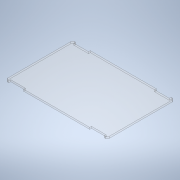
# Autodesk Inventor part: roof
Saved by Autodesk Inventor 2020 (Build 240168000, 168)
## iProperties
Created: 2020-03-02
Part Number: roof
Material: Polycarbonate, Clear
Document SubType Name: Modeling
Designer: n10208577
Density: 1.2 g/cm^3
Appearance: Polycarbonate - Clear
Author: n10208577
Autodesk Inventor part; units mm, degrees
ref_plane "YZ Plane" through (0, 0, 0) normal (1, 0, 0) x (0, 1, 0)
ref_plane "XZ Plane" through (0, 0, 0) normal (0, 1, 0) x (-1, 0, 0)
ref_plane "XY Plane" through (0, 0, 0) normal (0, 0, 1) x (1, 0, 0)
sketch "Sketch1" plane through (0, 0, 0) normal (0, 1, 0) x (-1, 0, 0)
  line L0 (25.1331, -7.9898) -> (138.1331, -7.9898)
  line L1 (-4.8669, 103.0102) -> (-4.8669, -4.9898)
  arc A0 (-4.8669, -4.9898) -> (-1.8669, -7.9898) centre (-1.8669, -4.9898) ccw
  line L2 (0.1331, -7.9898) -> (0.1331, -4.9898)
  line L3 (0.1331, -4.9898) -> (25.1331, -4.9898)
  line L4 (25.1331, -4.9898) -> (25.1331, -7.9898)
  line L5 (165.1331, -7.9898) -> (163.1331, -7.9898)
  line L6 (163.1331, -7.9898) -> (163.1331, -4.9898)
  line L7 (163.1331, -4.9898) -> (138.1331, -4.9898)
  line L8 (138.1331, -4.9898) -> (138.1331, -7.9898)
  line L9 (168.1331, -4.9898) -> (168.1331, 103.0102)
  arc A1 (165.1331, -7.9898) -> (168.1331, -4.9898) centre (165.1331, -4.9898) ccw
  arc A2 (168.1331, 103.0102) -> (165.1331, 106.0102) centre (165.1331, 103.0102) ccw
  line L10 (0.1331, -7.9898) -> (-1.8669, -7.9898)
  line L11 (25.1331, 106.0102) -> (138.1331, 106.0102)
  line L12 (0.1331, 106.0102) -> (0.1331, 103.0102)
  line L13 (0.1331, 103.0102) -> (25.1331, 103.0102)
  line L14 (25.1331, 103.0102) -> (25.1331, 106.0102)
  line L15 (165.1331, 106.0102) -> (163.1331, 106.0102)
  line L16 (163.1331, 106.0102) -> (163.1331, 103.0102)
  line L17 (163.1331, 103.0102) -> (138.1331, 103.0102)
  line L18 (138.1331, 103.0102) -> (138.1331, 106.0102)
  line L19 (0.1331, 106.0102) -> (-1.8669, 106.0102)
  arc A3 (-1.8669, 106.0102) -> (-4.8669, 103.0102) centre (-1.8669, 103.0102) ccw
  point P0 (0, 0)
  constraints: 40 end point, 8 point on circle, 4 centre point
extrude "Extrusion1" add sketch "Sketch1" along normal blind 3
body "Solid1"
